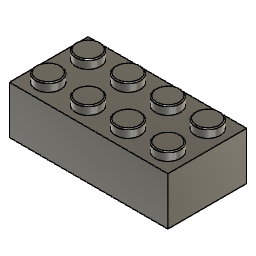
LEGO BRICK (Autodesk Fusion 360 design; units mm, degrees)
Autodesk Fusion 360 part; units mm, degrees
sketch "Sketch1" plane through (0, 0, 0) normal (1, 0, 0) x (0, 1, 0) in component "LEGO"
sketch "Sketch2" plane through (0, 0, 0) normal (0, 0, 1) x (1, 0, 0) in component "LEGO"
  line L0 (0, 0) -> (-31.8, 0)
  line L1 (-31.8, 0) -> (-31.8, -15.8)
  line L2 (-31.8, -15.8) -> (0, -15.8)
  line L3 (0, -15.8) -> (0, 0)
  dimension "d1" = 31.8
  dimension "d2" = 15.8
  constraint horizontal L0
  constraint vertical L1
  constraint horizontal L2
  constraint vertical L3
  constraint coincident L0.start L3.end
  measures "d1" distance of L0.start L0.end
  measures "d2" distance of L0.start L2.end
extrude "Extrude1" add sketch "Sketch2" along normal blind 9.6 in component "LEGO"
sketch "Sketch3" plane through (0, 0, 9.6) normal (0, 0, 1) x (-1, 0, 0) in component "LEGO"
  line L0 (0, 15.8) -> (0, 0)
  line L1 (0, 0) -> (31.8, 0)
  line L2 (31.8, 0) -> (31.8, 15.8)
  line L3 (31.8, 15.8) -> (0, 15.8)
  circle A0 centre (3.9, 11.9) radius 2.5
  dimension "d5" = 5
  dimension "d6" = 3.9
  dimension "d7" = 3.9
  measures "d5" diameter of A0
  measures "d6" distance of L3 A0.centre
  measures "d7" distance of L0 A0.centre
extrude "Extrude2" add sketch "Sketch3" along normal blind 1.7 contours A0 in component "LEGO"
pattern_linear "R-Pattern1" count 4 spacing 8 along (-1, 0, 0) count 2 spacing 8 along (0, 1, 0) of "Extrude2" in component "LEGO"
shell "Shell1" thickness 1.49 removed faces 1 at (-21.2, -10.5333, 0) in component "LEGO"
sketch "Sketch4" plane through (0, 0, 8.11) normal (0, 0, -1) x (1, 0, 0) in component "LEGO"
  circle A0 centre (-27.9, 3.9) radius 1.01
  circle A1 centre (-19.9, 3.9) radius 1.01
  circle A2 centre (-11.9, 3.9) radius 1.01
  circle A3 centre (-3.9, 3.9) radius 1.01
  circle A4 centre (-27.9, 11.9) radius 1.01
  circle A5 centre (-19.9, 11.9) radius 1.01
  circle A6 centre (-11.9, 11.9) radius 1.01
  circle A7 centre (-3.9, 11.9) radius 1.01
  line L0 (-1.49, 1.49) -> (-1.49, 14.31)
  line L1 (-1.49, 14.31) -> (-30.31, 14.31)
  line L2 (-30.31, 14.31) -> (-30.31, 1.49)
  line L3 (-30.31, 1.49) -> (-1.49, 1.49)
  line L4 (-19.9, 11.9) -> (-27.9, 3.9) construction
  circle A8 centre (-23.9, 7.9) radius 3.1016
  circle A9 centre (-23.9, 7.9) radius 2.1016
  dimension "d15" = -1
  constraint coincident A5.centre L4.start
  constraint coincident A0.centre L4.end
  constraint midpoint L4 A8.centre
extrude "Extrude3" add sketch "Sketch4" along normal blind 8.1 contours A8 in component "LEGO"
pattern_linear "R-Pattern2" count 3 spacing 8 along (1, 0, 0) of "Extrude3" in component "LEGO"
fillet "Fillet1" radius 0.2 8 edges at (-25.5692, -2.996, 11.3) (-17.5692, -2.996, 11.3) (-9.5692, -2.996, 11.3) (-1.5692, -2.996, 11.3) (-1.5692, -10.996, 11.3) (-9.5692, -10.996, 11.3) (-17.5692, -10.996, 11.3) (-25.5692, -10.996, 11.3) in component "LEGO"
fillet "Fillet2" radius 0.2 3 edges at (-10.7917, -6.7784, 0.01) (-18.7917, -6.7784, 0.01) (-26.7917, -6.7784, 0.01) in component "LEGO"
fillet "Fillet3" radius 0.2 3 edges at (-9.8594, -8.66, 0.01) (-17.8594, -8.66, 0.01) (-25.8594, -8.66, 0.01) in component "LEGO"
component "LEGO" placed x (1, 0, 0) y (0, 1, 0) z (0, 0, 1) at (0, 0, 0)
